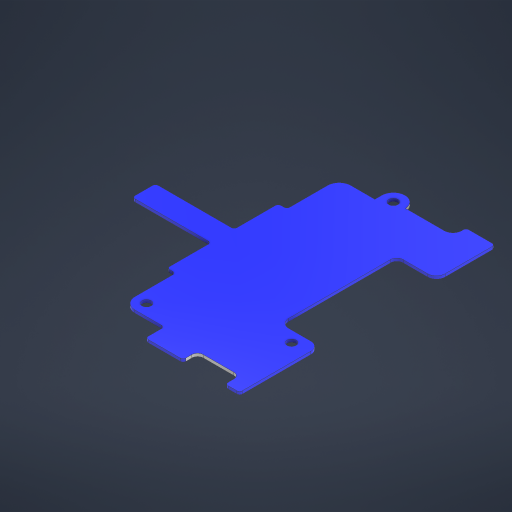
# Autodesk Inventor part: pcb
Saved by Autodesk Inventor 2024 (Build 280153000, 153)
## iProperties
Created: 2024-05-25
Part Number: pcb
Material: Generic
Document SubType Name: Modeling
Designer: Adam
Density: 1 g/cm^3
Appearance: Default
Author: Adam
Autodesk Inventor part; units mm, degrees
ref_plane "YZ Plane" through (0, 0, 0) normal (1, 0, 0) x (0, 1, 0)
ref_plane "XZ Plane" through (0, 0, 0) normal (0, 1, 0) x (-1, 0, 0)
ref_plane "XY Plane" through (0, 0, 0) normal (0, 0, 1) x (1, 0, 0)
ref_plane "Work Plane2" through (0, 1, 0) normal (0, 1, 0) x (1, 0, 0)
sketch "Sketch2" plane through (0, 1, 0) normal (0, 1, 0) x (1, 0, 0)
  line L0 (19.1771, -13.3933) -> (19.1771, 21.7206)
  arc A0 (-13.8229, -33.4026) -> (-9.8229, -37.4026) centre (-9.8229, -33.4026) ccw
  arc A1 (-9.8229, 36.9551) -> (-13.8229, 32.9551) centre (-9.8229, 32.9551) ccw
  circle A2 centre (2.4699, 39.3408) radius 1.55
  circle A3 centre (26.9336, -20.1907) radius 1.55
  circle A4 centre (-9.8229, -33.4026) radius 1.55
  line L1 (23.7927, 44.0538) -> (31.7927, 44.0538)
  line L2 (32.7927, 43.0538) -> (32.7927, 26.8418)
  line L3 (29.7927, 23.8418) -> (21.2983, 23.8418)
  line L4 (22.1771, -16.3933) -> (29.7927, -16.3933)
  line L5 (-17.8229, 3.7762) -> (-42.9549, 3.7762)
  line L6 (-43.9549, 2.7762) -> (-43.9549, -3.2238)
  line L7 (-42.9549, -4.2238) -> (-17.8229, -4.2238)
  line L8 (32.7927, -19.3933) -> (32.7927, -42.9467)
  line L9 (28.7927, -43.9467) -> (31.7927, -43.9467)
  line L10 (22.7927, 43.0538) -> (22.7927, 42.5538)
  arc A5 (23.7927, 44.0538) -> (22.7927, 43.0538) centre (23.7927, 43.0538) ccw
  arc A6 (32.7927, 43.0538) -> (31.7927, 44.0538) centre (31.7927, 43.0538) ccw
  arc A7 (31.7927, -43.9467) -> (32.7927, -42.9467) centre (31.7927, -42.9467) ccw
  arc A8 (27.7927, -42.9467) -> (28.7927, -43.9467) centre (28.7927, -42.9467) ccw
  arc A9 (29.7927, 23.8418) -> (32.7927, 26.8418) centre (29.7927, 26.8418) ccw
  arc A10 (19.7927, 39.5538) -> (22.7927, 42.5538) centre (19.7927, 42.5538) ccw
  arc A11 (19.1771, -13.3933) -> (22.1771, -16.3933) centre (22.1771, -13.3933) ccw
  arc A12 (32.7927, -19.3933) -> (29.7927, -16.3933) centre (29.7927, -19.3933) ccw
  arc A13 (21.2983, 23.8418) -> (19.1771, 21.7206) centre (21.2983, 21.7206) ccw
  arc A14 (-42.9549, 3.7762) -> (-43.9549, 2.7762) centre (-42.9549, 2.7762) ccw
  arc A15 (-43.9549, -3.2238) -> (-42.9549, -4.2238) centre (-42.9549, -3.2238) ccw
  line L11 (-13.8229, 32.9551) -> (-13.8229, 19.9551)
  line L12 (-14.8229, 18.9551) -> (-15.8229, 18.9551)
  line L13 (-16.8229, 17.9551) -> (-16.8229, 4.7762)
  line L14 (-13.8229, -33.4026) -> (-13.8229, -20.4026)
  line L15 (-14.8229, -19.4026) -> (-15.8229, -19.4026)
  line L16 (-16.8229, -18.4026) -> (-16.8229, -5.2238)
  arc A16 (-14.8229, 18.9551) -> (-13.8229, 19.9551) centre (-14.8229, 19.9551) ccw
  arc A17 (-15.8229, 18.9551) -> (-16.8229, 17.9551) centre (-15.8229, 17.9551) ccw
  arc A18 (-17.8229, 3.7762) -> (-16.8229, 4.7762) centre (-17.8229, 4.7762) ccw
  arc A19 (-16.8229, -5.2238) -> (-17.8229, -4.2238) centre (-17.8229, -5.2238) ccw
  arc A20 (-16.8229, -18.4026) -> (-15.8229, -19.4026) centre (-15.8229, -18.4026) ccw
  arc A21 (-13.8229, -20.4026) -> (-14.8229, -19.4026) centre (-14.8229, -20.4026) ccw
  arc A22 (2.4699, 43.3408) -> (-1.5298, 39.3918) centre (2.4699, 39.3408) ccw
  line L17 (-1.5298, 39.3918) -> (-1.5298, 36.9551)
  line L18 (-1.5298, 36.9551) -> (-9.8229, 36.9551)
  line L19 (12.2983, -43.9467) -> (1.2983, -43.9467)
  line L20 (0.2983, -42.9467) -> (0.2983, -38.4026)
  line L21 (-0.7017, -37.4026) -> (-9.8229, -37.4026)
  arc A23 (0.2983, -42.9467) -> (1.2983, -43.9467) centre (1.2983, -42.9467) ccw
  arc A24 (12.2983, -43.9467) -> (13.2983, -42.9467) centre (12.2983, -42.9467) ccw
  arc A25 (0.2983, -38.4026) -> (-0.7017, -37.4026) centre (-0.7017, -38.4026) ccw
  line L22 (19.7927, 39.5538) -> (8.4489, 39.5538)
  line L23 (27.7927, -42.9467) -> (27.7927, -40.9467)
  line L24 (25.7927, -38.9467) -> (15.2983, -38.9467)
  arc A26 (27.7927, -40.9467) -> (25.7927, -38.9467) centre (25.7927, -40.9467) ccw
  line L25 (13.2983, -42.9467) -> (13.2983, -40.9467)
  arc A27 (15.2983, -38.9467) -> (13.2983, -40.9467) centre (15.2983, -40.9467) ccw
  line L26 (8.4489, 39.5538) -> (6.4642, 39.5538)
  arc A28 (6.4642, 39.5538) -> (2.4699, 43.3408) centre (2.4699, 39.3408) ccw
  point P0 (0, 0)
  point P1 (19.1771, 23.8418)
  point P2 (22.7927, 44.0538)
  point P3 (32.7927, 44.0538)
  point P4 (32.7927, 23.8418)
  point P5 (32.7927, -16.3933)
  point P6 (32.7927, -43.9467)
  point P7 (25.9849, -16.3933)
  point P8 (19.1771, -16.3933)
  point P9 (-16.8229, 3.7762)
  point P10 (-16.8229, -4.2238)
  point P11 (30.2927, -43.9467)
  point P12 (-13.8229, 18.9551)
  point P13 (-16.8229, 18.9551)
  point P14 (-13.8229, -19.4026)
  point P15 (-16.8229, -19.4026)
  point P16 (13.2983, -43.9467)
  point P17 (0.2983, -43.9467)
  point P18 (0.2983, -37.4026)
  point P19 (27.7927, -38.9467)
  point P20 (27.7927, -42.9467)
  dimension "d13" = 3.1
  dimension "d15" = 3.1
  dimension "d26" = 1
  dimension "d27" = 3
  dimension "d30" = 3
  dimension "d32" = 1
  dimension "d33" = 20.212
  dimension "d36" = 14
  dimension "d37" = 3
  dimension "d38" = 14
  dimension "d39" = 3
  dimension "d40" = 1
  dimension "d41" = 36
  dimension "d42" = 13
  dimension "d43" = 1
  dimension "d45" = 3.7974
  dimension "d46" = 40.2351
  dimension "d47" = 88.0005
  dimension "d49" = 4
  dimension "d50" = 2
  dimension "d51" = 2
  dimension "d52" = 0.5
  constraints: 54 end point, 52 point on circle, 42 tangent, 33 point on line, 29 centre point, 13 equal radius, 10 perpendicular, 7 vertical, 4 horizontal, 2 coincident, 2 midpoint, 1 parallel
  measures "d13" diameter of A2
  measures "d15" diameter of A4
  measures "d26" radius of A5
  measures "d27" radius of A9
  measures "d30" radius of A11
  measures "d32" radius of A14
  measures "d33" distance between parallel lines of L3 L1
  measures "d36" distance of L11.start point (-13.823, 18.955)
  measures "d37" distance of point (-13.823, 18.955) point (-16.823, 18.955)
  measures "d38" distance of L14.start point (-13.823, -19.403)
  measures "d39" distance between parallel lines of L14 L16
  measures "d40" radius of A16
  measures "d41" distance between parallel lines of L13 L0
  measures "d42" distance of point (13.298, -43.947) point (0.298, -43.947)
  measures "d43" radius of A23
  measures "d45" distance from line of L4 A3.centre
  measures "d46" distance between parallel lines of L4 L3
  measures "d47" distance between parallel lines of L9 L1
  measures "d49" distance of L23.start point (27.793, -38.947)
  measures "d50" radius of A26
  measures "d51" radius of A27
  measures "d52" distance of L10.start L10.end
extrude "Extrusion2" add sketch "Sketch2" along normal blind 1
body "Solid2"
